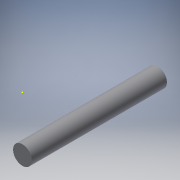
# Autodesk Inventor part: nema11_test
Saved by Autodesk Inventor 2019 (Build 230136000, 136)
## iProperties
Created: 2021-10-11
Part Number: nema11_test
Material: Generic
Document SubType Name: Modeling
Designer: Pokick
Density: 1 g/cm^3
Appearance: Default
Author: Pokick
Autodesk Inventor part; units mm, degrees
ref_plane "YZ Plane" through (0, 0, 0) normal (1, 0, 0) x (0, 1, 0)
ref_plane "XZ Plane" through (0, 0, 0) normal (0, 1, 0) x (-1, 0, 0)
ref_plane "XY Plane" through (0, 0, 0) normal (0, 0, 1) x (1, 0, 0)
sketch "Sketch1" plane through (0, 0, 0) normal (0, 0, 1) x (1, 0, 0)
  line L0 (0, 0) -> (14, 0) construction
  line L1 (14, 0) -> (-14, 0) construction
  line L2 (-14, 0) -> (-14, -22) construction
  line L3 (-14, -22) -> (14, -22) construction
  line L4 (14, -22) -> (14, 0) construction
  line L5 (0, 0) -> (0, -14.5) construction
  circle A0 centre (0, -14.5) radius 2 construction
  line L6 (-14, -28.5) -> (14, -28.5) construction
  line L7 (14, -28.5) -> (14, -0.5) construction
  line L8 (14, -0.5) -> (-14, -0.5) construction
  line L9 (-14, -0.5) -> (-14, -28.5) construction
  line L10 (-14, -28.5) -> (14, -0.5) construction
  line L11 (14, -28.5) -> (-14, -0.5) construction
  circle A1 centre (0, -14.5) radius 2.5
  dimension "d0" = 14
  dimension "d1" = 28
  dimension "d2" = 22
  dimension "d3" = 14.5
  dimension "d4" = 4
  dimension "d5" = 28
  dimension "d6" = 28
  dimension "d7" = 5
  constraints: 24 end point, 4 parallel, 3 horizontal, 2 centre point, 2 coincident, 2 midpoint, 2 perpendicular, 1 vertical
  measures "d0" distance of L0.start L0.end
  measures "d1" distance of L3.end L2.end
  measures "d2" distance of L2.end L1.end
  measures "d3" distance of L0.start L5.end
  measures "d4" diameter of A0
  measures "d5" distance of L8.end L7.end
  measures "d6" distance of L7.end L6.end
  measures "d7" diameter of A1
extrude "Extrusion1" add sketch "Sketch1" along normal blind 36
sketch "Sketch2" plane through (0, -14.5, 36) normal (0, 0, 1) x (1, 0, 0)
  point P0 (0, 14.5)
body "Solid1"
